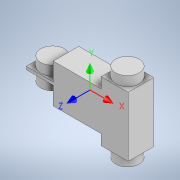
# Autodesk Inventor part: body
Saved by Autodesk Inventor 2020.2 (Build 242310000, 310)
## iProperties
Created: 2021-01-29
Part Number: body
Material: Generic
Document SubType Name: Modeling
Designer: DELL
Density: 1 g/cm^3
Appearance: Default
Author: DELL
Autodesk Inventor part; units mm, degrees
ref_plane "YZ Plane" through (0, 0, 0) normal (1, 0, 0) x (0, 1, 0)
ref_plane "XZ Plane" through (0, 0, 0) normal (0, 1, 0) x (-1, 0, 0)
ref_plane "XY Plane" through (0, 0, 0) normal (0, 0, 1) x (1, 0, 0)
sketch "Sketch1" plane through (0, 0, 0) normal (0, 0, 1) x (1, 0, 0)
  line L0 (-170, 5) -> (170, 5)
  line L1 (170, 5) -> (170, -5)
  line L2 (170, -5) -> (-170, -5)
  line L3 (-170, -5) -> (-170, 5)
  line L4 (-170, 5) -> (170, -5) construction
  line L5 (170, 5) -> (-170, -5) construction
  line L6 (-80, 65) -> (80, 65)
  line L7 (80, 65) -> (80, -65)
  line L8 (80, -65) -> (-80, -65)
  line L9 (-80, -65) -> (-80, 65)
  line L10 (-80, 65) -> (80, -65) construction
  line L11 (80, 65) -> (-80, -65) construction
  line L12 (-80, 125) -> (-80, -55)
  line L13 (170, 100) -> (80, 100)
  line L14 (80, 100) -> (80, -100)
  line L15 (80, -100) -> (170, -100)
  line L16 (170, -100) -> (170, 100)
  line L17 (170, 100) -> (80, -100) construction
  line L18 (80, 100) -> (170, -100) construction
  point P0 (0, 0)
  point P1 (0, 0)
  point P2 (80, -5)
  point P3 (80, 5)
  point P4 (125, 0)
  point P5 (0, 0)
  point P6 (125, 0)
  point P7 (170, 5)
  point P8 (80, 100)
  point P9 (170, -5)
  point P10 (-80, -5)
  point P11 (-80, 5)
  dimension "d0" = 10
  dimension "d1" = 340
  dimension "d2" = 160
  dimension "d3" = 130
  dimension "d13" = 200
  constraints: 38 end point, 9 midpoint, 6 parallel, 3 horizontal, 3 perpendicular, 2 point on line, 1 collinear, 1 horizontal alignment
  measures "d0" distance of L0.end L1.end
  measures "d1" distance of L0.start L0.end
  measures "d2" distance of L6.start L6.end
  measures "d3" distance between parallel lines of L6 L8
  measures "d13" distance of L15.end L13.start
extrude "Extrusion1" add sketch "Sketch1" along normal mid plane 85
sketch "Sketch2" plane through (0, 0, 0) normal (0, 1, 0) x (-1, 0, 0)
  circle A0 centre (-125, 0) radius 39.5
  circle A1 centre (125, 0) radius 39.5
  line L0 (0, 42.5) -> (0, -42.5) construction
  line L1 (170, 0) -> (-170, 0) construction
  line L2 (170, 0) -> (-170, 0) construction
  line L3 (170, -42.5) -> (170, 42.5) construction
  point P0 (0, 0)
  point P1 (0, 0)
  point P2 (0, 0)
  dimension "d7" = 79
  dimension "d8" = 250
  constraints: 6 end point, 3 midpoint, 2 centre point, 1 equal radius, 1 horizontal alignment, 1 perpendicular, 1 point on line, 1 symmetric about line
  measures "d7" diameter of A0
  measures "d8" distance of A0.centre A1.centre
extrude "Extrusion2" add sketch "Sketch2" against normal blind 32 from surface at -100 contours A0
extrude "Extrusion3" add sketch "Sketch2" against normal blind 32 from surface at -5 contours A1
mirror "Mirror1" about plane through (0, 0, 0) normal (0, 1, 0) of "Extrusion3", "Extrusion2"
body "Solid1"
